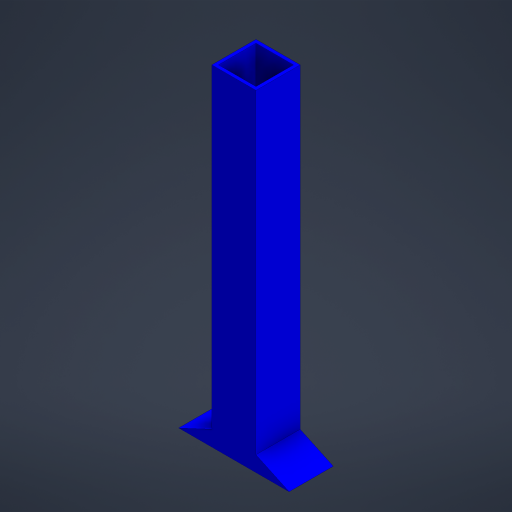
# Autodesk Inventor part: shock_absorber_holder
Saved by Autodesk Inventor 2024 (Build 280153000, 153)
## iProperties
Created: 2023-05-07
Part Number: shock_absorber_holder
Material: Типовые
Document SubType Name: Modeling
Designer: user
Density: 1 g/cm^3
Appearance: По умолчанию
Author: user
Autodesk Inventor part; units mm, degrees
ref_plane "YZ Plane" through (0, 0, 0) normal (1, 0, 0) x (0, 1, 0)
ref_plane "XZ Plane" through (0, 0, 0) normal (0, 1, 0) x (-1, 0, 0)
sketch "Эскиз1" plane through (0, 0, 0) normal (0, 0, 1) x (1, 0, 0)
  line L0 (0, 0) -> (20, 0)
  line L1 (20, 0) -> (20, 20)
  line L2 (20, 20) -> (0, 20)
  line L3 (0, 20) -> (0, 0)
  line L4 (1.5, 1.5) -> (18.5, 1.5)
  line L5 (18.5, 1.5) -> (18.5, 18.5)
  line L6 (18.5, 18.5) -> (1.5, 18.5)
  line L7 (1.5, 18.5) -> (1.5, 1.5)
  point P0 (10, 18.5)
  point P1 (10, 20)
  point P2 (18.5, 10)
  point P3 (20, 10)
  dimension "d0" = 20
  dimension "d1" = 1.5
  constraints: 16 end point, 4 midpoint, 4 parallel, 4 perpendicular, 2 horizontal, 1 horizontal alignment, 1 vertical alignment
  measures "d0" distance of L1.end L2.end
  measures "d1" horizontal distance of L1.end L5.end
extrude "Выдавливание1" add sketch "Эскиз1" along normal blind 150
sketch "Эскиз3" plane through (0, 20, 0) normal (0, 1, 0) x (1, 0, 0)
  line L0 (0, 0) -> (0, -150) projected
  line L1 (0, -7) -> (-15, 0)
  line L2 (-15, 0) -> (0, 0)
  line L3 (0, 0) -> (0, -7)
  line L4 (0, -7) -> (0, 0)
  dimension "d4" = 15
  dimension "d5" = 7
  constraints: 8 end point, 2 perpendicular, 1 collinear, 1 point on line
  measures "d4" distance of L1.end L0.start
  measures "d5" distance of L0.start L1.start
extrude "Выдавливание2" add sketch "Эскиз3" against normal up to surface (20 mm away)
ref_plane "РабПлоскость1" through (10, 0, 150) normal (-1, 0, 0) x (0, 0, 1)
mirror "Зеркальное отражение1" about plane through (10, 0, 150) normal (-1, 0, 0) of "Выдавливание2"
